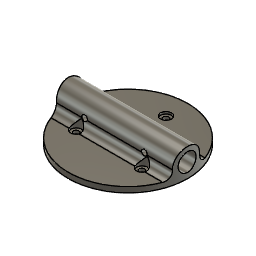
gaseta EMF platina v9 (Autodesk Fusion 360 design; units mm, degrees)
Autodesk Fusion 360 part; units mm, degrees
sketch "Boceto1" plane through (0, 0, 0) normal (0, 1, 0) x (1, 0, 0)
  circle A0 centre (0, 0) radius 55
  dimension "d47" = 110
  constraint coincident A0.centre origin
  measures "d47" diameter of A0
extrude "Extruir1" add sketch "Boceto1" along normal blind 5 contours A0 picked at (-30.929263, -6.680934)
ref_plane "PlanoDeObra1" through (0, 0, 0) normal (1, 0, 0) x (0, 1, 0)
sketch "Boceto2" plane through (0, 0, 0) normal (1, 0, 0) x (0, 0, -1)
  circle A0 centre (-0.000043, 13.25) radius 5
  circle A1 centre (-0.000043, 13.25) radius 8.25
  circle A2 centre (-0.000043, 13.25) radius 12.5
  point P0 (0, 5)
  dimension "d11" = 16.5
  dimension "d43" = 10
  dimension "d50" = 25
  dimension "d61" = 8.25
  dimension "d66" = 4.25
  constraint concentric A0 A1
  constraint concentric A1 A2
  measures "d11" diameter of A1
  measures "d43" diameter of A0
  measures "d50" diameter of A2
  measures "d66" distance of A1 A2
extrude "Extruir2" add sketch "Boceto2" along normal mid plane 110 contours A2 picked at (11.006037, 12.219124)
sketch "Boceto3" plane through (0, 0, 0) normal (0, 1, 0) x (1, 0, 0)
  circle A0 centre (0, 0) radius 55
  circle A1 centre (0, 0) radius 100
  constraint coincident A0.centre A1.centre
  constraint concentric A0 A1
extrude "Extruir3" cut sketch "Boceto3" along normal blind 30 contours A1 picked at (84.422926, -7.700517)
fillet "Empalme1" radius 7 1 edges at (0, 5, 9.390863)
fillet "Empalme2" radius 7 1 edges at (0, 5, -9.390777)
sketch "Boceto4" plane through (0, 0, 0) normal (0, 0, 1) x (1, 0, 0)
  circle A0 centre (-27.5, 13.25) radius 3.5
  circle A1 centre (27.5, 13.25) radius 3.5
  circle A2 centre (-27.5, 13.25) radius 2.5
  circle A3 centre (27.5, 13.25) radius 2.5
  line L0 (55, 21.5) -> (55, 5)
  circle A4 centre (55, 13.25) radius 0.338832
  line L1 (55, 13.25) -> (-55, 13.25)
  line L2 (55, 13.25) -> (27.5, 13.25)
  line L3 (-55, 13.25) -> (-27.5, 13.25)
  point P0 (55, 21.5)
  point P1 (55, 5)
  dimension "d20" = 7
  dimension "d21" = 7
  dimension "d48" = 5
  dimension "d49" = 5
  dimension "d62" = 16.5
  dimension "d63" = 110
  dimension "d64" = 27.5
  dimension "d65" = 27.5
  constraint concentric A0 A2
  constraint concentric A1 A3
  constraint coincident P0 L0.start
  constraint coincident P1 L0.end
  constraint midpoint L0 A4.centre
  constraint coincident A4.centre L1.start
  constraint horizontal L1
  constraint perpendicular L0 L2
  constraint coincident A1.centre A3.centre
  constraint parallel L1 L3
  constraint coincident A0.centre A2.centre
  measures "d20" diameter of A0
  measures "d21" diameter of A1
  measures "d48" diameter of A2
  measures "d49" diameter of A3
  measures "d62" distance of P0 P1
  measures "d63" distance of A4.centre L1.end
  measures "d64" distance of A4.centre A1.centre
  measures "d65" distance of L1.end A0.centre
extrude "Extruir4" cut sketch "Boceto4" along normal mid plane 35 contours A2 L1 L3 | A2 L1 L3 picked at (-29.157359, 13.374202) picked at (-25.842641, 13.125798)
extrude "Extruir5" cut sketch "Boceto4" along normal mid plane 42 contours A3 L1 L2 | A3 L1 L2 picked at (25.952882, 13.857199) picked at (25.842641, 13.125798)
sketch "Boceto5" plane through (0, 0, 0) normal (0, 1, 0) x (1, 0, 0)
  circle A0 centre (-40, 0) radius 6
  dimension "d79" = 12
  measures "d79" diameter of A0
extrude "Extruir6" cut sketch "Boceto5" along normal blind 10.2 contours A0 picked at (-38.418778, -1.864711)
sketch "Boceto6" plane through (0, 5, 0) normal (0, 1, 0) x (-1, 0, 0)
  circle A0 centre (0, -35) radius 2.5
  circle A1 centre (0, 0) radius 35
  circle A2 centre (30.310889, 17.5) radius 2.5
  circle A3 centre (-30.310889, 17.5) radius 2.5
  arc A4 (51.442306, 19.459938) -> (-51.442306, 19.459938) centre (0, 0) ccw
  line L0 (-51.442306, 19.459938) -> (51.442306, 19.459938)
  line L1 (51.442338, -19.459852) -> (-51.442338, -19.459852)
  arc A5 (-51.442338, -19.459852) -> (51.442338, -19.459852) centre (0, 0) ccw
  dimension "d28" = 5
  dimension "d34" = 35
  dimension "d35" = 70
  dimension "d37" = 360
  constraint coincident A1.centre A4.centre
  constraint coincident A0.centre A1
  measures "d28" diameter of A0
  measures "d34" distance of A1.centre A0.centre
  measures "d35" diameter of A1
extrude "Extruir7" cut sketch "Boceto6" along normal blind -20 and the other way blind -40 contours A0 A1 | A0 A1 | A1 A3 L0 | A1 A3 L0 | A1 A2 L0 | A1 A2 L0 | A1 A3 L0 | A1 A3 L0 | A1 A2 L0 | A1 A2 L0 picked at (-0.014883, -35.826584) picked at (0.060861, -34.162276) picked at (-31.078198, 17.823341) picked at (-29.64418, 16.979171) picked at (29.639874, 16.985693) picked at (31.109435, 17.755416) picked at (-30.845296, 19.524284) picked at (-28.89414, 19.478534) picked at (28.89414, 19.478534) picked at (30.845296, 19.524284)
sketch "Boceto7" plane through (0, 0, 0) normal (0, 1, 0) x (1, 0, 0)
  circle A0 centre (0, 35.000001) radius 7.5
  circle A1 centre (-30.31089, -17.5) radius 7.5
  circle A2 centre (30.31089, -17.5) radius 7.5
  dimension "d44" = 15
  dimension "d46" = 360
  measures "d44" diameter of A0
sketch "Boceto8" plane through (0, 5, 0) normal (0, 1, 0) x (-1, 0, 0)
  line L0 (31.86287, 19.459938) -> (51.442306, 19.459938)
  arc A0 (51.442306, 19.459938) -> (-51.442306, 19.459938) centre (0, 0) ccw
  circle A1 centre (-30.310889, 17.5) radius 2.5
  line L1 (-29.040719, 15.3) -> (-27.770548, 17.5)
  line L2 (-27.770548, 17.5) -> (-29.040719, 19.7)
  line L3 (-29.040719, 19.7) -> (-31.58106, 19.7)
  line L4 (-31.58106, 19.7) -> (-32.85123, 17.5)
  line L5 (-32.85123, 17.5) -> (-31.58106, 15.3)
  line L6 (-31.58106, 15.3) -> (-29.040719, 15.3)
  arc A2 (31.86287, 19.459938) -> (28.758908, 19.459938) centre (30.310889, 17.5) ccw
  line L7 (-51.442306, 19.459938) -> (-31.86287, 19.459938)
  arc A3 (-28.758908, 19.459938) -> (-31.86287, 19.459938) centre (-30.310889, 17.5) ccw
  line L8 (-28.758908, 19.459938) -> (28.758908, 19.459938)
  point P0 (-30.310889, 17.5)
  dimension "d57" = 5
  dimension "d58" = 2.2
  measures "d57" diameter of A1
sketch "Boceto9" plane through (0, 5, 0) normal (0, 1, 0) x (-1, 0, 0)
  arc A0 (31.86287, 19.459938) -> (28.758908, 19.459938) centre (30.310889, 17.5) ccw
  line L0 (31.86287, 19.459938) -> (51.442306, 19.459938)
  arc A1 (51.442306, 19.459938) -> (-51.442306, 19.459938) centre (0, 0) ccw
  line L1 (-51.442306, 19.459938) -> (-31.86287, 19.459938)
  arc A2 (-28.758908, 19.459938) -> (-31.86287, 19.459938) centre (-30.310889, 17.5) ccw
  line L2 (-28.758908, 19.459938) -> (28.758908, 19.459938)
  circle A3 centre (0, -35.000001) radius 3.5
  circle A4 centre (30.31089, 17.5) radius 3.5
  circle A5 centre (-30.31089, 17.5) radius 3.5
  circle A6 centre (30.310889, 17.5) radius 5
  circle A7 centre (-30.310889, 17.5) radius 5
  circle A8 centre (0, -35) radius 5
  line L3 (29.86811, 12.474335) -> (53.566697, 12.474335)
  dimension "d67" = 7
  dimension "d69" = 360
  dimension "d74" = 10
  dimension "d76" = 360
  dimension "d78" = 10
  dimension "d80" = 7
  constraint concentric A0 A6
  measures "d67" diameter of A3
  measures "d74" diameter of A6
  measures "d78" diameter of A7
  measures "d80" diameter of A4
extrude "Extruir10" cut sketch "Boceto9" along normal blind 7 and the other way blind 2 contours A0 L0 L2 A4 | A0 L0 L2 A4 | L0 L2 A4 A6 | L0 L2 A4 A6 | L1 L2 A5 A7 | L1 L2 A5 A7 | L1 A2 L2 A5 | L1 A2 L2 A5 | A3 | A8 picked at (30.225769, 17.643068) picked at (30.535058, 20.653029) picked at (26.642064, 20.089784) picked at (26.048775, 18.913637) picked at (-34.573004, 18.913637) picked at (-26.642064, 20.089784) picked at (-30.396009, 17.643068) picked at (-30.535058, 20.653029) picked at (0.901775, -35.912137) picked at (-1.868466, -30.919149)
